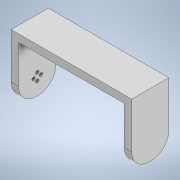
# Autodesk Inventor part: tilt_output_bracket
Saved by Autodesk Inventor 2022 (Build 260153000, 153)
## iProperties
Created: 2022-01-23
Part Number: tilt_output_bracket
Material: Generic
Document SubType Name: Modeling
Designer: Mlees
Density: 1 g/cm^3
Appearance: Default
Author: Mlees
Autodesk Inventor part; units mm, degrees
ref_plane "YZ Plane" through (0, 0, 0) normal (1, 0, 0) x (0, 1, 0)
ref_plane "XZ Plane" through (0, 0, 0) normal (0, 1, 0) x (-1, 0, 0)
ref_plane "XY Plane" through (0, 0, 0) normal (0, 0, 1) x (1, 0, 0)
sketch "Sketch1" plane through (0, 0, 0) normal (0, 1, 0) x (-1, 0, 0)
  line L0 (0, 0) -> (130, 0)
  line L1 (130, 0) -> (130, -40)
  line L2 (130, -40) -> (0, -40)
  line L3 (0, -40) -> (0, 0)
  dimension "d0" = 130
  dimension "d1" = 40
  constraints: 8 end point, 2 parallel, 1 horizontal, 1 perpendicular
  measures "d0" distance of L1.end L2.end
  measures "d1" distance of L0.end L1.end
extrude "Extrusion1" add sketch "Sketch1" along normal blind 50
sketch "Sketch3" plane through (-130, 0, 0) normal (0, 0, 1) x (1, 0, 0)
  line L0 (130, 0) -> (0, 0) projected
  line L1 (0, 0) -> (8, 0)
  line L2 (8, 0) -> (8, 42)
  line L3 (130, 50) -> (0, 50) projected
  line L4 (122, 0) -> (122, 42)
  line L5 (8, 42) -> (122, 42)
  line L6 (8, 0) -> (122, 0)
  dimension "d8" = 8
  dimension "d9" = 42
  constraints: 10 end point, 1 collinear, 1 horizontal, 1 perpendicular, 1 point on line
  measures "d8" distance of L0.end L1.end
  measures "d9" distance of L1.end L2.end
extrude "Extrusion3" cut sketch "Sketch3" against normal through all
sketch "Sketch4" plane through (0, 0, 0) normal (0, -1, 0) x (1, 0, 0)
  line L0 (-130, -40) -> (-130, 0) projected
  line L1 (-8, -40) -> (-122, -40) projected
  line L2 (-130, 0) -> (-122, 0)
  line L3 (-122, 0) -> (-122, -40)
  line L4 (-122, -40) -> (-130, -40)
  line L5 (-130, -40) -> (-130, 0)
  line L6 (-8, 0) -> (0, 0)
  line L7 (0, 0) -> (0, -40)
  line L8 (0, -40) -> (-8, -40)
  line L9 (-8, -40) -> (-8, 0)
  constraints: 16 end point, 4 parallel, 2 horizontal, 2 perpendicular
extrude "Extrusion4" add sketch "Sketch4" along normal blind 18
sketch "Sketch7" plane through (-130, 50, -40) normal (-1, 0, 0) x (0, 0, 1)
  line L0 (40, -68) -> (0, -68) projected
  line L1 (20, -68) -> (20, -50)
  circle A0 centre (20, -46) radius 1.75
  circle A1 centre (16, -50) radius 1.75
  circle A2 centre (20, -54) radius 1.75
  circle A3 centre (24, -50) radius 1.75
  point P0 (40, -50)
  dimension "d23" = 18
  dimension "d25" = 3.5
  dimension "d28" = 360
  constraints: 4 centre point, 2 end point, 1 coincident, 1 midpoint, 1 vertical, 9 other
  measures "d23" distance of L1.start L1.end
  measures "d25" diameter of A0
extrude "Extrusion6" cut sketch "Sketch7" against normal up to surface (8 mm away)
fillet "Fillet1" radius 18.75 4 edges at (-126, -18, -40) (-126, -18, 0) (-4, -18, 0) (-4, -18, -40)
sketch "Sketch8" plane through (0, 50, 0) normal (1, 0, 0) x (0, 0, -1)
  line L0 (16, -50) -> (24, -50)
  line L1 (20, -54) -> (20, -46)
  circle A0 centre (20, -50) radius 6.4
  point P0 (0, -50)
  dimension "d33" = 12.8
  constraints: 4 end point, 1 centre point, 1 horizontal, 1 midpoint, 1 vertical
  measures "d33" diameter of A0
extrude "Extrusion7" add sketch "Sketch8" against normal blind 15
body "Solid1"
